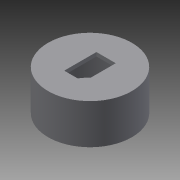
# Autodesk Inventor part: per_base
Saved by Autodesk Inventor 2015 (Build 190159000, 159)
## iProperties
Created: 2014-10-20
Part Number: per_base
Material: Generic
Document SubType Name: Modeling
Designer: ericd_000
Density: 1 g/cm^3
Appearance: Default
Author: ericd_000
Autodesk Inventor part; units mm, degrees
ref_plane "YZ Plane" through (0, 0, 0) normal (1, 0, 0) x (0, 1, 0)
ref_plane "XZ Plane" through (0, 0, 0) normal (0, 1, 0) x (-1, 0, 0)
ref_plane "XY Plane" through (0, 0, 0) normal (0, 0, 1) x (1, 0, 0)
sketch "Sketch1" plane through (0, 0, 0) normal (0, 0, 1) x (1, 0, 0)
  circle A0 centre (0, 0) radius 65
  dimension "d0" = 130
  constraints: 1 centre point, 1 coincident
  measures "d0" diameter of A0
extrude "Extrusion1" add sketch "Sketch1" along normal blind 6
sketch "Sketch2" plane through (0, 0, 6) normal (0, 0, 1) x (1, 0, 0)
  circle A0 centre (0, 0) radius 65
  circle A1 centre (0, 0) radius 65 projected
  circle A2 centre (0, 0) radius 59
  dimension "d3" = 6
  constraints: 2 centre point, 2 concentric, 1 coincident
  measures "d3" radial gap between concentric circles of A0 A2
extrude "Extrusion2" add sketch "Sketch2" along normal blind 50
sketch "Sketch3" plane through (0, 0, 56) normal (0, 0, 1) x (1, 0, 0)
  circle A0 centre (0, 0) radius 65
  constraints: 1 centre point, 1 coincident
extrude "Extrusion3" add sketch "Sketch3" along normal blind 6
sketch "Sketch4" plane through (0, 0, 62) normal (0, 0, 1) x (1, 0, 0)
  line L0 (-15, -25) -> (15, -25)
  line L1 (15, -25) -> (15, 25)
  line L2 (15, 25) -> (-15, 25)
  line L3 (-15, 25) -> (-15, -25)
  line L4 (0, 0) -> (-15, 0) construction
  point P0 (0, -25)
  dimension "d9" = 50
  dimension "d10" = 30
  constraints: 10 end point, 3 midpoint, 2 horizontal, 2 parallel, 1 horizontal alignment, 1 perpendicular, 1 vertical alignment
  measures "d9" distance of L0.end L1.end
  measures "d10" distance of L1.end L2.end
extrude "Extrusion4" cut sketch "Sketch4" against normal blind 6
sketch "Sketch5" plane through (0, 0, 62) normal (0, 0, 1) x (1, 0, 0)
  line L0 (15, 25) -> (25, 25)
  line L1 (25, 25) -> (25, -5)
  line L2 (25, -5) -> (15, -5)
  line L3 (15, -5) -> (15, 25)
  point P0 (0, 0)
  dimension "d13" = 30
  dimension "d14" = 10
  constraints: 8 end point, 2 parallel, 1 horizontal, 1 perpendicular
  measures "d13" distance of L0.end L1.end
  measures "d14" distance of L1.end L2.end
extrude "Extrusion5" [suppressed]
sketch "Sketch6" plane through (15, -25, 56) normal (-1, 0, 0) x (0, 0, 1)
  circle A0 centre (33, 23.5) radius 1
  circle A1 centre (33, 6.5) radius 1
  line L0 (36, 30) -> (36, 0) projected
  line L1 (33, 23.5) -> (33, 6.5) construction
  point P0 (-56, 25)
  point P1 (36, 15)
  point P2 (33, 15)
  dimension "d17" = 17
  dimension "d19" = 2
  dimension "d20" = 2
  dimension "d21" = 3
  constraints: 2 centre point, 2 end point, 2 midpoint, 1 horizontal alignment, 1 vertical, 1 vertical alignment
  measures "d17" distance of L1.end L1.start
  measures "d19" diameter of A1
  measures "d20" diameter of A0
  measures "d21" distance from line of L0 L1.start
extrude "Extrusion6" [suppressed]
body "Solid1"
